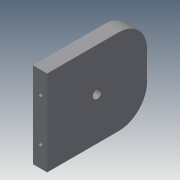
# Autodesk Inventor part: stojan_rameno
Saved by Autodesk Inventor 2013 (Build 170138000, 138)
## iProperties
Created: 2013-05-25
Part Number: stojan_rameno
Material: Generic
Document SubType Name: Modeling
Designer: idle-rug
Density: 1 g/cm^3
Author: idle-rug
Autodesk Inventor part; units mm, degrees
ref_plane "YZ Plane" through (0, 0, 0) normal (1, 0, 0) x (0, 1, 0)
ref_plane "XZ Plane" through (0, 0, 0) normal (0, 1, 0) x (-1, 0, 0)
ref_plane "XY Plane" through (0, 0, 0) normal (0, 0, 1) x (1, 0, 0)
sketch "Sketch1" plane through (0, 0, 0) normal (1, 0, 0) x (0, 1, 0)
  circle A0 centre (0, 0) radius 25
  line L0 (35, -50) -> (-35, -50)
  line L1 (-35, -50) -> (-35, 50)
  line L2 (-35, 50) -> (35, 50)
  line L3 (35, 50) -> (35, -50)
  line L4 (35, -50) -> (-35, 50) construction
  line L5 (-35, -50) -> (35, 50) construction
  circle A1 centre (0, 0) radius 3
  dimension "d0" = 50
  dimension "d1" = 70
  dimension "d2" = 100
  dimension "d3" = 6
  constraints: 12 end point, 2 centre point, 2 coincident, 2 midpoint, 2 parallel, 1 horizontal, 1 perpendicular
  measures "d0" diameter of A0
  measures "d1" distance of L1.end L2.end
  measures "d2" distance of L2.end L0.start
  measures "d3" diameter of A1
extrude "Extrusion1" add sketch "Sketch1" along normal blind 10 contours A0 | L0 L1 L2 L3
fillet "Fillet1" radius 50 2 edges at (5, 35, 50) (5, 35, -50)
sketch "Sketch2" plane through (10, 0, 0) normal (1, 0, 0) x (0, 0, -1)
  arc A0 (50, -15) -> (-50, -15) centre (0, -15) ccw projected
  line L0 (-50, -15) -> (-50, -35) projected
  line L1 (-50, -35) -> (50, -35) projected
  line L2 (50, -35) -> (50, -15) projected
  circle A1 centre (0, 0) radius 3 projected
  line L3 (50, 35) -> (-50, 35)
  line L4 (-50, 35) -> (-50, -35)
  line L5 (-50, -35) -> (50, -35)
  line L6 (50, -35) -> (50, 35)
  line L7 (50, 35) -> (-50, -35) construction
  line L8 (-50, 35) -> (50, -35) construction
  constraints: 12 end point, 2 midpoint, 2 parallel, 1 horizontal, 1 perpendicular
extrude "Extrusion2" add sketch "Sketch2" against normal blind 10 contours A0 L3 L6 | A0 L4 L3
sketch "Sketch3" plane through (10, 0, 0) normal (1, 0, 0) x (0, 0, -1)
  line L0 (-50, 35) -> (-50, -35) projected
  line L1 (-50, -35) -> (50, -35) projected
  line L2 (50, -35) -> (50, 35) projected
  line L3 (50, 35) -> (-50, 35) projected
  circle A0 centre (0, 0) radius 3 projected
  line L4 (30, 35) -> (-30, 35)
  line L5 (-30, 35) -> (-30, -35)
  line L6 (-30, -35) -> (30, -35)
  line L7 (30, -35) -> (30, 35)
  line L8 (30, 35) -> (-30, -35) construction
  line L9 (-30, 35) -> (30, -35) construction
  dimension "d9" = 60
  constraints: 12 end point, 2 midpoint, 2 parallel, 1 horizontal, 1 perpendicular, 1 point on line
  measures "d9" distance of L6.end L5.end
extrude "Extrusion3" cut sketch "Sketch3" against normal blind 10 contours L3 L5 L1 L0 | L3 L2 L1 L7
fillet "Fillet2" radius 20 2 edges at (5, 35, 30) (5, 35, -30)
sketch "Sketch4" plane through (0, -35, -30) normal (0, -1, 0) x (1, 0, 0)
  line L0 (0, 0) -> (10, 0) projected
  line L1 (0, 0) -> (0, 60) projected
  line L2 (5, 0) -> (5, 15)
  line L3 (5, 15) -> (5, 45)
  circle A0 centre (5, 15) radius 1.5
  circle A1 centre (5, 45) radius 1.5
  point P0 (0, 30)
  dimension "d13" = 15
  dimension "d14" = 30
  dimension "d15" = 3
  dimension "d16" = 3
  constraints: 4 end point, 2 centre point, 2 coincident, 1 collinear, 1 midpoint, 1 parallel
  measures "d13" distance of L2.start L2.end
  measures "d14" distance of L2.end L3.end
  measures "d15" diameter of A0
  measures "d16" diameter of A1
extrude "Extrusion4" cut sketch "Sketch4" against normal blind 10
sketch "Sketch5" plane through (10, 0, 0) normal (1, 0, 0) x (0, 0, -1)
  circle A0 centre (0, 0) radius 3 projected
  line L0 (-30, -35) -> (30, -35) projected
  circle A1 centre (0, 0) radius 25
  line L1 (0, -35) -> (-50, -35)
  line L2 (-50, -35) -> (50, -35)
  line L3 (21.4679, 12.8113) -> (50, -35)
  line L4 (-50, -35) -> (-21.4679, 12.8113)
  dimension "d19" = 50
  dimension "d20" = 50
  dimension "d21" = 100
  constraints: 8 end point, 2 point on circle, 2 point on line, 1 centre point, 1 coincident, 1 midpoint, 1 tangent
  measures "d19" diameter of A1
  measures "d20" distance of L1.start L1.end
  measures "d21" distance of L1.end L2.end
extrude "Extrusion5" add sketch "Sketch5" along normal blind 10
sketch "Sketch6" plane through (0, 0, 0) normal (-1, 0, 0) x (0, 0, 1)
  arc A0 (-10, 35) -> (-30, 15) centre (-10, 15) ccw projected
  line L0 (-30, 15) -> (-30, -35) projected
  line L1 (-30, -35) -> (30, -35) projected
  line L2 (30, -35) -> (30, 15) projected
  arc A1 (30, 15) -> (10, 35) centre (10, 15) ccw projected
  line L3 (10, 35) -> (-10, 35) projected
  circle A2 centre (0, 0) radius 3 projected
extrude "Extrusion6" cut sketch "Sketch6" against normal blind 10
sketch "Sketch7" plane through (10, 0, 0) normal (-1, 0, 0) x (0, 0, 1)
  circle A0 centre (0, 0) radius 3 projected
  line L0 (-21.4679, 12.8113) -> (-50, -35) projected
  line L1 (50, -35) -> (-50, -35) projected
  line L2 (50, -35) -> (21.4679, 12.8113) projected
  arc A1 (21.4679, 12.8113) -> (-21.4679, 12.8113) centre (0, 0) ccw projected
body "Solid1"
